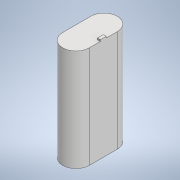
# Autodesk Inventor part: Battery
Saved by Autodesk Inventor 2020.2 (Build 242310000, 310)
## iProperties
Created: 2020-03-13
Part Number: Battery
Material: Generic
Document SubType Name: Modeling
Designer: linus
Density: 1 g/cm^3
Appearance: Default
Author: linus
Autodesk Inventor part; units mm, degrees
ref_plane "YZ Plane" through (0, 0, 0) normal (1, 0, 0) x (0, 1, 0)
ref_plane "XZ Plane" through (0, 0, 0) normal (0, 1, 0) x (-1, 0, 0)
ref_plane "XY Plane" through (0, 0, 0) normal (0, 0, 1) x (1, 0, 0)
sketch "Sketch1" plane through (0, 0, 0) normal (0, 1, 0) x (-1, 0, 0)
  line L0 (0, 18.5) -> (0, 18.5)
  line L1 (-9, 9.5) -> (-9, -9.5)
  line L2 (0, -18.5) -> (0, -18.5)
  line L3 (9, -9.5) -> (9, 9.5)
  arc A0 (9, 9.5) -> (0, 18.5) centre (0, 9.5) ccw
  arc A1 (0, -18.5) -> (9, -9.5) centre (0, -9.5) ccw
  arc A2 (-9, -9.5) -> (0, -18.5) centre (0, -9.5) ccw
  arc A3 (0, 18.5) -> (-9, 9.5) centre (0, 9.5) ccw
  point P0 (0, 0)
  point P1 (-9, -18.5)
  point P2 (-9, 18.5)
  point P3 (9, -18.5)
  point P4 (0, -18.5)
  dimension "d0" = 18
  dimension "d1" = 37
  dimension "d2" = 18.5
  dimension "d3" = 9
  dimension "d4" = 9
  constraints: 8 end point, 8 point on circle, 8 tangent, 6 point on line, 4 centre point, 3 equal radius, 2 parallel, 1 horizontal, 1 perpendicular
  measures "d0" distance of point (-9, -18.5) point (9, -18.5)
  measures "d1" distance of point (-9, 18.5) point (-9, -18.5)
  measures "d2" distance from line of point (0, 0) L0
  measures "d3" distance from line of point (0, 0) L1
  measures "d4" radius of A0
extrude "Extrusion1" add sketch "Sketch1" along normal blind 69
sketch "Sketch2" plane through (0, 69, 0) normal (0, 1, 0) x (1, 0, 0)
  line L0 (9, -9.5) -> (9, 9.5) projected
  line L1 (9, 2) -> (7, 2)
  line L2 (7, 2) -> (7, -2)
  line L3 (7, -2) -> (9, -2)
  line L4 (9, -2) -> (9, 2)
  point P0 (0, 0)
  dimension "d7" = 2
  dimension "d8" = 4
  dimension "d9" = 2
  constraints: 8 end point, 2 parallel, 1 horizontal, 1 perpendicular, 1 point on line
  measures "d7" distance of L3.end L2.end
  measures "d8" distance of L2.end L1.end
  measures "d9" distance from line of point (0, 0) L3
extrude "Extrusion2" add sketch "Sketch2" along normal blind 1
equation "\"d2\" = 0.5 * d1"
equation "\"d3\" = 0.5 * d0"
equation "\"d8\" = 2 * d7"
equation "\"d9\" = 0.5 * d8"
body "Solid1"
